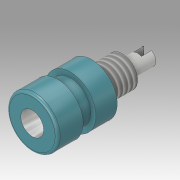
# Autodesk Inventor part: banana_plug_recepticle
Saved by Autodesk Inventor 2019.3 (Build 233278000, 278)
## iProperties
Created: 2019-03-22
Part Number: banana_plug_recepticle
Material: Generic
Document SubType Name: Modeling
Designer: Dave
Density: 1 g/cm^3
Appearance: Default
Author: Dave
Autodesk Inventor part; units mm, degrees
ref_plane "YZ Plane" through (0, 0, 0) normal (1, 0, 0) x (0, 1, 0)
ref_plane "XZ Plane" through (0, 0, 0) normal (0, 1, 0) x (-1, 0, 0)
ref_plane "XY Plane" through (0, 0, 0) normal (0, 0, 1) x (1, 0, 0)
sketch "Sketch1" plane through (0, 0, 0) normal (0, 0, 1) x (1, 0, 0)
  circle A0 centre (0, 0) radius 5
  dimension "d0" = 10
  constraints: 1 centre point, 1 coincident
  measures "d0" diameter of A0
extrude "Extrusion1" add sketch "Sketch1" along normal blind 5
sketch "Sketch2" plane through (0, 0, 0) normal (0, 0, -1) x (-1, 0, 0)
  circle A0 centre (0, 0) radius 5 projected
  circle A1 centre (0, 0) radius 4
  dimension "d3" = 8
  constraints: 1 centre point, 1 coincident
  measures "d3" diameter of A1
extrude "Extrusion2" add sketch "Sketch2" along normal blind 2.5 contours A1
sketch "Sketch3" plane through (0, 0, 5) normal (0, 0, 1) x (1, 0, 0)
  circle A0 centre (0, 0) radius 5 projected
  circle A1 centre (0, 0) radius 2.25
  dimension "d6" = 4.5
  constraints: 1 centre point, 1 coincident
  measures "d6" diameter of A1
extrude "Extrusion3" cut sketch "Sketch3" against normal through all contours A1
fillet "Fillet1" radius 0.5 1 edges at (-5, 0, 5)
sketch "Sketch4" plane through (0, 0, -2.5) normal (0, 0, -1) x (-1, 0, 0)
  circle A0 centre (0, 0) radius 2.25 projected
  circle A1 centre (0, 0) radius 2.25 projected
  circle A2 centre (0, 0) radius 4 projected
  circle A3 centre (0, 0) radius 4 projected
  circle A4 centre (0, 0) radius 5 projected
  circle A5 centre (0, 0) radius 5
  constraints: 1 centre point, 1 coincident, 1 concentric
extrude "Extrusion4" add sketch "Sketch4" along normal blind 4.2 contours A2 | A4
sketch "Sketch5" plane through (0, 0, -6.7) normal (0, 0, -1) x (-1, 0, 0)
  circle A0 centre (0, 0) radius 2.25 projected
  circle A1 centre (0, 0) radius 3
  dimension "d12" = 6
  constraints: 1 centre point, 1 coincident
  measures "d12" diameter of A1
extrude "Extrusion5" add sketch "Sketch5" along normal blind 7 contours A0 | A1
sketch "Sketch6" plane through (0, 0, -13.7) normal (0, 0, -1) x (-1, 0, 0)
  circle A0 centre (0, 0) radius 3 projected
  circle A1 centre (0, 0) radius 1.6
  dimension "d15" = 3.2
  constraints: 1 centre point, 1 coincident
  measures "d15" diameter of A1
extrude "Extrusion6" add sketch "Sketch6" along normal blind 4 contours A1
sketch "Sketch7" plane through (0, 0, -17.7) normal (0, 0, -1) x (-1, 0, 0)
  line L0 (0.75, -1.6) -> (-0.75, -1.6)
  line L1 (-0.75, -1.6) -> (-0.75, 1.6)
  line L2 (-0.75, 1.6) -> (0.75, 1.6)
  line L3 (0.75, 1.6) -> (0.75, -1.6)
  circle A0 centre (0, 0) radius 1.6 projected
  point P0 (0, -1.6)
  point P1 (0.75, 0)
  dimension "d18" = 1.5
  constraints: 8 end point, 2 midpoint, 2 parallel, 1 horizontal, 1 horizontal alignment, 1 perpendicular, 1 tangent, 1 vertical alignment
  measures "d18" distance of L0.start L0.end
extrude "Extrusion7" cut sketch "Sketch7" against normal blind 2 contours L0 A0 L3 | L0 L1 A0 | A0 L1 L3 | A0 L2 L3 | L1 L2 A0
chamfer "Chamfer1" distance 1.4 distance2 1 1 edges at (3, 0, -13.7) measured on face at (2.5, 0, -13.7)
thread "Thread1" size "M6x1" class "6g" standard "ANSI Metric M Profile" full length
body "Solid1"
